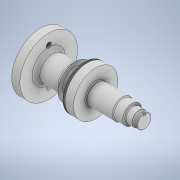
# Autodesk Inventor part: 69. Блок шестерен промежуточного вала
Saved by Autodesk Inventor 2021 (Build 250183000, 183)
## iProperties
Created: 2021-03-22
Part Number: 69. Блок шестерен промежуточного вала
Material: Типовые
Document SubType Name: Modeling
Designer: Данил
Density: 1 g/cm^3
Appearance: По умолчанию
Author: Данил
Autodesk Inventor part; units mm, degrees
ref_plane "YZ Plane" through (0, 0, 0) normal (1, 0, 0) x (0, 1, 0)
ref_plane "XY Plane" through (0, 0, 0) normal (0, 0, 1) x (1, 0, 0)
sketch "Эскиз1" plane through (0, 0, 0) normal (0, 0, 1) x (1, 0, 0)
  line L0 (-128.5, 0) -> (128.5, 0)
  line L1 (128.5, 0) -> (128.5, -15.5)
  line L2 (127.5, -16.5) -> (116.5, -16.5)
  line L3 (127.5, -16.5) -> (128.5, -15.5)
  line L4 (116.5, -16.5) -> (116.5, -17.5)
  line L5 (116.5, -17.5) -> (102.5, -17.5)
  line L6 (102.3557, -17.25) -> (99.5, -17.25)
  line L7 (102.5, -17.5) -> (102.3557, -17.25)
  line L8 (102.3557, -17.25) -> (102.3557, 0) construction
  line L9 (99.5, -17.25) -> (99.5, -22.5)
  line L10 (99.5, -22.5) -> (79, -22.5)
  line L11 (77, -24.5) -> (17.366, -24.5)
  arc A0 (79, -22.5) -> (77, -24.5) centre (79, -24.5) ccw
  line L12 (17.366, -24.5) -> (16.5, -24)
  arc A1 (16.5, -24) -> (13.5, -25.7321) centre (15.5, -25.7321) ccw
  line L13 (13.5, -25.7321) -> (13.5, -52.283)
  line L14 (13.5, -52.283) -> (-6.5, -52.283)
  line L15 (-6.5, -52.283) -> (-6.5, -43.5)
  line L16 (-6.5, -43.5) -> (-11.5, -43.5)
  line L17 (-11.5, -43.5) -> (-11.5, -51.134)
  line L18 (-11.5, -51.134) -> (-12, -52)
  line L19 (-12, -52) -> (-12, -68.35)
  line L20 (-12, -68.35) -> (-34.5, -68.35)
  line L21 (-34.5, -68.35) -> (-34.5, -41)
  line L22 (-45.5, -30) -> (-88.5, -30)
  arc A2 (-34.5, -41) -> (-45.5, -30) centre (-45.5, -41) ccw
  line L23 (-97.5, -39) -> (-97.5, -81.1)
  arc A3 (-88.5, -30) -> (-97.5, -39) centre (-88.5, -39) ccw
  line L24 (-97.5, -81.1) -> (-117, -81.1)
  line L25 (-117, -81.1) -> (-117, -66.5)
  line L26 (-117, -66.5) -> (-117, -66.5)
  line L27 (-110, -59.5) -> (-110, -24.5)
  arc A4 (-117, -66.5) -> (-110, -59.5) centre (-117, -59.5) ccw
  line L28 (-110, -24.5) -> (-112.5, -22)
  line L29 (-112.5, -22) -> (-112.5, -17.25)
  line L30 (-112.5, -17.25) -> (-115.3557, -17.25)
  line L31 (-115.3557, -17.25) -> (-115.5, -17.5)
  line L32 (-115.5, -17.5) -> (-127.5, -17.5)
  line L33 (-128.5, -16.5) -> (-128.5, 0)
  line L34 (-127.5, -17.5) -> (-128.5, -16.5)
  point P0 (0, 0)
  point P1 (0, 0)
  point P2 (128.5, -16.5)
  point P3 (-128.5, -17.5)
  dimension "d0" = 257
  dimension "d1" = 33
  dimension "d2" = 1
  dimension "d3" = 45
  dimension "d4" = 35
  dimension "d5" = 34.5
  dimension "d6" = 30
  dimension "d7" = 3
  dimension "d8" = 17
  dimension "d9" = 29
  dimension "d10" = 45
  dimension "d11" = 2
  dimension "d12" = 49
  dimension "d14" = 22.5
  dimension "d15" = 2
  dimension "d16" = 0.5
  dimension "d17" = 30
  dimension "d18" = 86
  dimension "d19" = 104.566
  dimension "d20" = 20
  dimension "d21" = 87
  dimension "d22" = 5
  dimension "d23" = 11
  dimension "d24" = 136.7
  dimension "d25" = 0.5
  dimension "d26" = 30
  dimension "d27" = 104
  dimension "d28" = 22.5
  dimension "d29" = 60
  dimension "d30" = 9
  dimension "d31" = 162.2
  dimension "d32" = 19.5
  dimension "d33" = 7
  dimension "d36" = 7
  dimension "d37" = 133
  dimension "d38" = 44
  dimension "d39" = 35
  dimension "d40" = 212
  dimension "d41" = 216.5
  dimension "d42" = 30
  dimension "d43" = 34.5
  dimension "d44" = 3
  dimension "d45" = 45
  dimension "d46" = 1
  dimension "d47" = 45
  constraints: 70 end point, 11 perpendicular, 10 point on circle, 9 tangent, 8 vertical, 7 horizontal, 6 point on line, 5 centre point, 2 coincident, 2 parallel, 1 midpoint, 1 vertical alignment, 3 other
  measures "d0" distance of L0.start L0.end
  measures "d1" diameter of L2 L0
  measures "d2" distance of L2.start point (128.5, -16.5)
  measures "d3" angle of L2 L3
  measures "d4" diameter of L5 L0
  measures "d5" diameter of L6 L0
  measures "d6" angle of L8 L7
  measures "d7" horizontal distance of L5.end L6.end
  measures "d8" distance from line of L4 L6.end
  measures "d9" distance from line of L1 L6.end
  measures "d10" diameter of L10 L0
  measures "d11" radius of A0
  measures "d12" diameter of L11 L0
  measures "d14" distance from line of L9 A0.end
  measures "d15" radius of A1
  measures "d16" distance from line of L11 L12.end
  measures "d17" angle of L11 L12
  measures "d18" distance between parallel lines of L9 L13
  measures "d19" diameter of L14 L0
  measures "d20" distance of L13.end L14.end
  measures "d21" diameter of L16 L0
  measures "d22" distance of L15.end L16.end
  measures "d23" radius of A2
  measures "d24" diameter of L20 L0
  measures "d25" horizontal distance of L18.end L17.end
  measures "d26" angle of L17 L18
  measures "d27" diameter of L18.end L0
  measures "d28" distance of L19.end L20.end
  measures "d29" diameter of L22 L0
  measures "d30" radius of A3
  measures "d31" diameter of L24 L0
  measures "d32" distance of L23.end L24.end
  measures "d33" radius of A4
  measures "d36" distance between parallel lines of L25 L27
  measures "d37" diameter of L25.end L0
  measures "d38" diameter of L28.end L0
  measures "d39" diameter of L32 L0
  measures "d40" distance between parallel lines of L9 L29
  measures "d41" distance between parallel lines of L9 L25
  measures "d42" angle of L29 L31
  measures "d43" diameter of L30 L0
  measures "d44" distance from line of L29 L31.end
  measures "d45" angle of L27 L28
  measures "d46" distance of L32.end point (-128.5, -17.5)
  measures "d47" angle of L32 L34
revolve "Вращение1" add sketch "Эскиз1" angle 360 about axis through (-128.5, 0, 0) along (1, 0, 0)
ref_plane "РабПлоскость1" through (0, 16.5, 0) normal (0, 1, 0) x (-1, 0, 0)
sketch "Эскиз2" plane through (0, 16.5, 0) normal (0, 1, 0) x (-1, 0, 0)
  line L0 (-128.5, -15.5) -> (-128.5, 15.5) projected
  line L1 (-123.5, -2.5) -> (-128.5, -2.5)
  line L2 (-128.5, -2.5) -> (-128.5, 2.5)
  line L3 (-128.5, 2.5) -> (-123.5, 2.5)
  line L4 (-123.5, 2.5) -> (-123.5, -2.5)
  point P0 (0, 0)
  point P1 (-123.5, 0)
  point P2 (-128.5, 0)
  point P3 (-128.5, 2.5)
  dimension "d50" = 5
  constraints: 8 end point, 3 midpoint, 2 parallel, 2 perpendicular, 1 horizontal, 1 horizontal alignment
  measures "d50" distance of L1.start L1.end
thread "Резьба1" size "M33x1" class "6g" standard "ISO Metric profile" length 9
extrude "Выдавливание1" cut sketch "Эскиз2" against normal blind 5
sketch "Эскиз3" plane through (-110, 0, 0) normal (-1, 0, 0) x (0, 0, 1)
  circle A0 centre (0, 0) radius 43 construction
  circle A1 centre (0, 43) radius 6
  circle A2 centre (0, -43) radius 6
  dimension "d55" = 86
  dimension "d56" = 12
  constraints: 3 centre point, 2 point on circle, 2 vertical alignment, 1 coincident, 1 equal radius
  measures "d55" diameter of A0
  measures "d56" diameter of A1
extrude "Выдавливание2" cut sketch "Эскиз3" against normal blind 34
sketch "Эскиз4" plane through (0, 0, 0) normal (0, 1, 0) x (-1, 0, 0)
  line L0 (117, -34) -> (117, 34) construction
  line L1 (112.5, -22) -> (112.5, 22) projected
  line L2 (117, -34) -> (117, -19)
  line L3 (117, -19) -> (108.5, -19)
  line L4 (108.5, -19) -> (99.8397, -34)
  line L5 (117, -66.5) -> (117, 66.5) projected
  line L6 (117, -34) -> (99.8397, -34)
  line L7 (97.5, -81.1) -> (97.5, 81.1) projected
  point P0 (0, 0)
  point P1 (117, 0)
  dimension "d59" = 68
  dimension "d64" = 4
  dimension "d65" = 30
  dimension "d66" = 60
  constraints: 10 end point, 2 midpoint, 1 horizontal, 1 horizontal alignment, 1 perpendicular, 1 point on line, 1 vertical
  measures "d59" distance of L0.start L0.end
  measures "d64" distance from line of L1 L3.end
  measures "d65" diameter of L3 L6
  measures "d66" angle of L6 L4
revolve "Вращение2" cut sketch "Эскиз4" angle 360 about axis through (-117, 0, -34) along (1, 0, 0)
mirror "Зеркальное отражение1" about plane through (0, 0, 0) normal (0, 0, 1) of "Вращение2"
sketch "Эскиз5" plane through (0, 0, 0) normal (0, 0, 1) x (1, 0, 0)
  line L0 (-128.5, 16.5) -> (-128.5, -16.5) projected
  line L1 (-128.5, 0) -> (0, 0)
  line L2 (-117, 81.1) -> (-117, -81.1) projected
  line L3 (-97.5, 81.1) -> (-97.5, -81.1) projected
  line L4 (-117, 81.1) -> (-97.5, 81.1)
  line L5 (-97.5, 81.1) -> (-97.5, 68)
  line L6 (-97.5, 68) -> (-117, 68)
  line L7 (-117, 68) -> (-117, 81.1)
  dimension "d68" = 136
  constraints: 10 end point, 2 horizontal, 2 parallel, 1 midpoint, 1 perpendicular, 1 point on line
  measures "d68" diameter of L6 L1
revolve "Вращение3" cut sketch "Эскиз5" angle 360 about axis through (-128.5, 0, 0) along (1, 0, 0) contours L2 L4 L3 L6
sketch "Эскиз6" plane through (0, 0, 0) normal (0, 0, 1) x (1, 0, 0)
  line L0 (-128.5, 16.5) -> (-128.5, -16.5) projected
  line L1 (-128.5, 0) -> (0, 0)
  line L2 (-34.5, 68.35) -> (-34.5, -68.35) projected
  line L3 (-12, 68.35) -> (-12, -68.35) projected
  line L4 (-34.5, 68.35) -> (-12, 68.35)
  line L5 (-12, 68.35) -> (-12, 30.5)
  line L6 (-12, 30.5) -> (-34.5, 30.5)
  line L7 (-34.5, 30.5) -> (-34.5, 68.35)
  dimension "d70" = 61
  constraints: 10 end point, 2 horizontal, 2 parallel, 1 midpoint, 1 perpendicular, 1 point on line
  measures "d70" diameter of L6 L1
revolve "Вращение4" cut sketch "Эскиз6" angle 360 about axis through (-128.5, 0, 0) along (1, 0, 0) contours L2 L4 L3 L6
